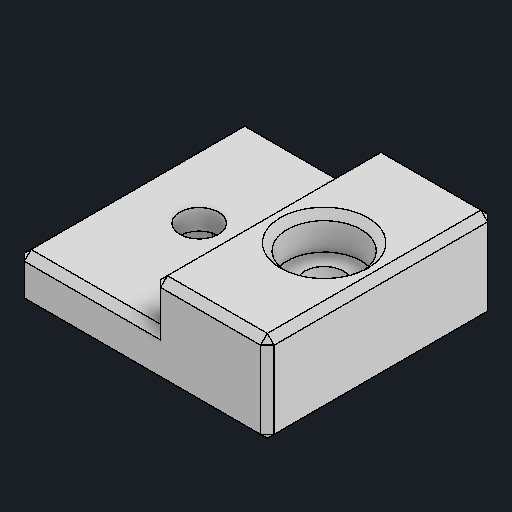
# Autodesk Inventor part: Part2
Saved by Autodesk Inventor 2026.2 (Build 302298000, 298)
## iProperties
Created: 2026-07-19
Part Number: Part2
Material: Generic
Document SubType Name: Modeling
Designer: JoshuaEah
Density: 1 g/cm^3
Appearance: Default
Author: JoshuaEah
Autodesk Inventor part; units mm, degrees
ref_plane "YZ Plane" through (0, 0, 0) normal (1, 0, 0) x (0, 1, 0)
ref_plane "XZ Plane" through (0, 0, 0) normal (0, 1, 0) x (-1, 0, 0)
ref_plane "XY Plane" through (0, 0, 0) normal (0, 0, 1) x (1, 0, 0)
sketch "Sketch1" plane through (0, 0, 0) normal (0, 1, 0) x (-1, 0, 0)
  line L0 (0, 0) -> (-22, 0)
  line L1 (-22, 0) -> (-22, -20)
  line L2 (-22, -20) -> (0, -20)
  line L3 (0, -20) -> (0, 0)
  line L4 (-12, -20) -> (-12, 0)
  point P0 (-17, -10)
  point P1 (-22, -10)
  point P2 (-6, -10)
  point P3 (0, -10)
  dimension "d0" = 20
  dimension "d5" = 12
  dimension "d7" = 5
  dimension "d8" = 5
  dimension "d25" = 6
  constraints: 10 end point, 2 horizontal alignment, 2 midpoint, 2 parallel, 2 perpendicular, 2 point on line, 1 coincident, 1 horizontal
  measures "d0" distance of L2.end L0.start
  measures "d5" distance between parallel lines of L4 L3
  measures "d7" distance from line of L4 point (-17, -10)
  measures "d8" distance from line of L1 point (-17, -10)
  measures "d25" distance from line of L3 point (-6, -10)
extrude "Extrusion1" add sketch "Sketch1" against normal blind 4
hole "Hole2" at (6, 0, -10) direction (0, -1, 0) diameter 3.4036 end through all clearance for "Socket Head Cap Screw" size "M3" standard "Ansi Metric M Profile"
sketch "Sketch3" plane through (0, -4, 0) normal (0, -1, 0) x (1, 0, 0)
  circle A0 centre (6, -10) radius 1.7018 construction
  line L0 (9.1754, -10) -> (7.5877, -12.75)
  line L1 (7.5877, -12.75) -> (4.4123, -12.75)
  line L2 (4.4123, -12.75) -> (2.8246, -10)
  line L3 (2.8246, -10) -> (4.4123, -7.25)
  line L4 (4.4123, -7.25) -> (7.5877, -7.25)
  line L5 (7.5877, -7.25) -> (9.1754, -10)
  dimension "d33" = 5.5
  constraints: 12 end point, 1 coincident, 1 horizontal, 13 other
  measures "d33" distance between parallel lines of L1 L4
extrude "Extrusion4" cut sketch "Sketch3" against normal blind 2.2
extrude "Extrusion2" add sketch "Sketch1" along normal blind 4 contours L4 L2 L1 L0
sketch "Sketch2" plane through (0, 4, 0) normal (0, 1, 0) x (1, 0, 0)
  point P0 (17, 10)
hole "Hole1" at (17, 4, -10) direction (0, -1, 0) diameter 3.4036 end through all counterbore diameter 6.5024 counterbore depth 2.9972 clearance for "Socket Head Cap Screw" size "M3" standard "Ansi Metric M Profile"
chamfer "Chamfer1" distance 0.6 angle 45 18 edges at (6, 0, -20) (12, 2, -20) (17, 4, -20) (22, 4, -10) (17, 4, 0) (12, 2, 0) (6, 0, 0) (0, -2, 0) (22, 0, 0) (22, 0, -20) (11, -4, -20) (22, -4, -10) (11, -4, 0) (0, -4, -10) (0, -2, -20) (17, 4, -13.2512) (0, 0, -10) (12, 4, -10)
equation "\"d8\" = d7"
equation "\"d25\" = 0.5 * d5"
body "Solid1"
